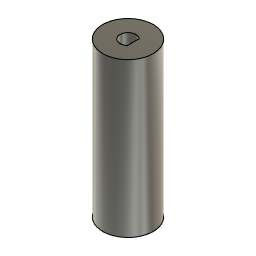
Connector Fusion360 (Autodesk Fusion 360 design; units mm, degrees)
Autodesk Fusion 360 part; units mm, degrees
sketch "Sketch1" plane through (0, 0, 0) normal (0, 0, 1) x (1, 0, 0)
  circle A0 centre (0, 0) radius 4.75
  dimension "d1" = 9.5
  constraint coincident A0.centre origin
  measures "d1" diameter of A0
extrude "Extrude1" add sketch "Sketch1" along normal blind 35
sketch "Sketch2" plane through (0, 0, 35) normal (0, 0, 1) x (-1, 0, 0)
  circle A0 centre (0, 0) radius 4.75
  arc A1 (-1, -1.118) -> (-1, 1.118) centre (0, 0) ccw
  line L0 (-1, -1.118) -> (-1, 1.118)
  constraint coincident A0.centre A1.centre
extrude "Extrude2" cut sketch "Sketch2" against normal blind 12 contours A1 L0
sketch "Sketch3" plane through (0, 0, 0) normal (0, 0, -1) x (1, 0, 0)
  circle A0 centre (0, 0) radius 4.75
  line L0 (2.75, 1.25) -> (-2.75, 1.25)
  line L1 (-2.75, 1.25) -> (-2.75, -1.25)
  line L2 (-2.75, -1.25) -> (2.75, -1.25)
  line L3 (2.75, -1.25) -> (2.75, 1.25)
  dimension "d9" = 5.5
  dimension "d10" = 2.5
  constraint horizontal L0
  constraint vertical L1
  constraint horizontal L2
  constraint vertical L3
  measures "d9" distance of L0.start L0.end
  measures "d10" distance of L0.start L2.end
extrude "Extrude3" cut sketch "Sketch3" against normal blind 18 contours L0 L1 L2 L3
extrude "Extrude4" cut 1 faces at (-0.9167, -0.4167, 18) along direction (0, 0, 1) blind 4
extrude "Extrude5" cut 1 faces at (0.1183, 2.4122, 0) along direction (0, 0, 1) blind 5
extrude "Extrude6" cut 1 faces at (0.1183, 2.4122, 5) along direction (0, 0, 1) blind 1
